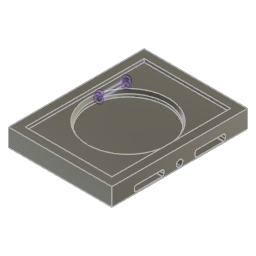
Plantillas_Taladrado (Autodesk Fusion 360 design; units mm, degrees)
Autodesk Fusion 360 part; units mm, degrees
note: some values were not read from the file. Set by a fixed rule: which sketch regions a step uses.
(part 1 of 4)
sketch "Boceto1" plane through (0, 0, 0) normal (0, 0, 1) x (1, 0, 0)
  line L0 (-350.383, -160) -> (-534, -160)
  line L1 (-455, -160) -> (-485, -160)
  line L2 (-349.3477, -167.8637) -> (-490.0029, -205.5522)
  line L3 (-513.132, -233.222) -> (-328.2758, -207.9962)
  line L4 (-333.1284, -237.9253) -> (-317, -237.9253) construction
  line L5 (246.2643, -265.6288) -> (-3.7357, -265.6288)
  line L6 (-3.7357, -235.6288) -> (246.2643, -235.6288)
  line L7 (246.2643, -235.6288) -> (246.2643, -265.6288)
  line L8 (-3.7357, -265.6288) -> (-3.7357, -235.6288)
  line L9 (-340.8744, -224.4717) -> (-532.4471, -275.8034)
  line L10 (-350.383, -160) -> (-534, -160)
  line L11 (-349.3477, -167.8637) -> (-490.0029, -205.5522)
  arc A0 (-334.1839, -233.9864) -> (-329.0577, -237.6835) centre (-329.3542, -232.6923) ccw
  line L12 (-517.6728, -197.507) -> (-517.6728, -229.2587)
  arc A1 (-496.8802, -195.3406) -> (-501.0926, -192.3911) centre (-500.7439, -196.3758) ccw
  line L13 (-326.1408, -237.5102) -> (-329.0577, -237.6835)
  line L14 (-497.7489, -192.0985) -> (-478.0528, -192.0985) construction
  line L15 (-501.0926, -192.3911) -> (-514.0215, -193.5222)
  arc A2 (-335.9754, -227.3001) -> (-340.8744, -224.4717) centre (-339.8392, -228.3354) ccw
  arc A3 (-534, -160) -> (-540, -166) centre (-534, -166) ccw
  line L16 (-497.7489, -192.0985) -> (-478.0528, -192.0985) construction
  line L17 (-334.1839, -233.9864) -> (-335.9754, -227.3001)
  arc A4 (-322.6085, -212.6538) -> (-328.2758, -207.9962) centre (-327.5997, -212.9503) ccw
  arc A5 (-326.1408, -237.5102) -> (-321.4461, -232.2225) centre (-326.4373, -232.519) ccw
  line L18 (-517.6728, -197.507) -> (-517.6728, -229.2587)
  circle A6 centre (-463, -175) radius 2.1
  arc A7 (-534, -160) -> (-540, -166) centre (-534, -166) ccw
  arc A8 (-349.3477, -167.8637) -> (-350.383, -160) centre (-350.383, -164) ccw
  arc A9 (-540, -270.0079) -> (-532.4471, -275.8034) centre (-534, -270.0079) ccw
  arc A10 (-335.9754, -227.3001) -> (-340.8744, -224.4717) centre (-339.8392, -228.3354) ccw
  arc A11 (-334.1839, -233.9864) -> (-329.0577, -237.6835) centre (-329.3542, -232.6923) ccw
  line L19 (-320, -160) -> (-304.7526, -160) construction
  line L20 (-494.9019, -202.7237) -> (-496.8802, -195.3406)
  line L21 (-540, -166) -> (-540, -270.0079)
  line L22 (-494.9019, -202.7237) -> (-496.8802, -195.3406)
  arc A12 (-494.9019, -202.7237) -> (-490.0029, -205.5522) centre (-491.0382, -201.6884) ccw
  line L23 (-322.6085, -212.6538) -> (-321.4461, -232.2225)
  line L24 (-501.0926, -192.3911) -> (-514.0215, -193.5222)
  arc A13 (-322.6085, -212.6538) -> (-328.2758, -207.9962) centre (-327.5997, -212.9503) ccw
  line L25 (-326.1408, -237.5102) -> (-329.0577, -237.6835)
  arc A14 (-514.0215, -193.5222) -> (-517.6728, -197.507) centre (-513.6728, -197.507) ccw
  arc A15 (-517.6728, -229.2587) -> (-513.132, -233.222) centre (-513.6728, -229.2587) ccw
  arc A16 (-494.9019, -202.7237) -> (-490.0029, -205.5522) centre (-491.0382, -201.6884) ccw
  arc A17 (-326.1408, -237.5102) -> (-321.4461, -232.2225) centre (-326.4373, -232.519) ccw
  line L26 (-322.6085, -212.6538) -> (-321.4461, -232.2225)
  arc A18 (-349.3477, -167.8637) -> (-350.383, -160) centre (-350.383, -164) ccw
  line L27 (-540, -166) -> (-540, -270.0079)
  arc A19 (-540, -270.0079) -> (-532.4471, -275.8034) centre (-534, -270.0079) ccw
  arc A20 (-496.8802, -195.3406) -> (-501.0926, -192.3911) centre (-500.7439, -196.3758) ccw
  circle A21 centre (-477, -175) radius 2.1
  arc A22 (-517.6728, -229.2587) -> (-513.132, -233.222) centre (-513.6728, -229.2587) ccw
  arc A23 (-514.0215, -193.5222) -> (-517.6728, -197.507) centre (-513.6728, -197.507) ccw
  line L28 (-513.132, -233.222) -> (-328.2758, -207.9962)
  line L29 (-340.8744, -224.4717) -> (-532.4471, -275.8034)
  line L30 (-334.1839, -233.9864) -> (-335.9754, -227.3001)
  line L31 (-525, -725) -> (-702.3195, -725)
  line L32 (1232.2, -850) -> (1286.175, -850)
  line L33 (-525, -547.6805) -> (-525, -573.0805)
  circle A24 centre (-525, -876.9195) radius 2.1
  circle A25 centre (-525, -573.0805) radius 2.1
  line L34 (263.0875, -557.9) -> (432.907, -557.9)
  line L35 (-525, -725) -> (-525, -902.3195)
  line L36 (0, -850) -> (53.975, -850)
  arc A26 (1023.0875, -697.7343) -> (828.975, -850) centre (1030.5875, -907.1583) ccw
  line L37 (248.0875, -627.75) -> (248.0875, -557.9)
  line L38 (432.907, -557.9) -> (263.0875, -557.9)
  line L39 (1030.5875, -627.75) -> (1023.0875, -627.75)
  line L40 (-347.6805, -725) -> (-373.0805, -725)
  line L41 (-525, -725) -> (-347.6805, -725)
  line L42 (1286.175, -850) -> (1207.907, -557.9)
  line L43 (775, -850) -> (853.268, -557.9)
  line L44 (263.0875, -557.9) -> (432.907, -557.9)
  line L45 (-347.6805, -725) -> (-296.8805, -725)
  line L46 (1038.0875, -627.75) -> (1038.0875, -697.7343)
  circle A27 centre (-373.0805, -725) radius 2.1
  line L47 (457.2, -850) -> (511.175, -850)
  circle A28 centre (-525, -725) radius 228.1195
  line L48 (511.175, -850) -> (510, -850)
  line L49 (511.175, -850) -> (457.2, -850)
  circle A29 centre (-676.9195, -725) radius 2.1
  line L50 (-702.3195, -725) -> (-676.9195, -725)
  line L51 (1030.5875, -627.75) -> (1038.0875, -627.75)
  arc A30 (457.2, -850) -> (53.975, -850) centre (255.5875, -907.1583) ccw
  line L52 (775, -850) -> (828.975, -850)
  line L53 (0, -850) -> (53.975, -850)
  line L54 (1286.175, -850) -> (1285, -850)
  line L55 (1207.907, -557.9) -> (1030.5875, -557.9)
  line L56 (0, -850) -> (78.268, -557.9)
  line L57 (263.0875, -557.9) -> (263.0875, -627.75)
  line L58 (1232.2, -850) -> (1286.175, -850)
  arc A31 (1232.2, -850) -> (1038.0875, -697.7343) centre (1030.5875, -907.1583) ccw
  line L59 (775, -850) -> (828.975, -850) construction
  line L60 (511.175, -850) -> (432.907, -557.9)
  line L61 (457.2, -850) -> (511.175, -850)
  line L62 (511.175, -850) -> (432.907, -557.9)
  line L63 (1286.175, -850) -> (1207.907, -557.9)
  line L64 (853.268, -557.9) -> (1207.907, -557.9)
  line L65 (-347.6805, -725) -> (-355.9463, -725)
  line L66 (1023.0875, -627.75) -> (1023.0875, -697.7343)
  line L67 (1286.175, -850) -> (1232.2, -850)
  line L68 (0, -850) -> (53.975, -850)
  line L69 (0, -850) -> (78.268, -557.9)
  line L70 (0, -850) -> (53.975, -850) construction
  line L71 (78.268, -557.9) -> (248.0875, -557.9)
  line L72 (853.268, -557.9) -> (1207.907, -557.9)
  line L73 (-525, -725) -> (-525, -547.6805)
  line L74 (78.268, -557.9) -> (248.0875, -557.9)
  line L75 (-525, -902.3195) -> (-525, -876.9195)
  line L76 (775, -850) -> (828.975, -850)
  line L77 (775, -850) -> (828.975, -850)
  line L78 (263.0875, -627.75) -> (248.0875, -627.75)
  line L79 (775, -850) -> (853.268, -557.9)
  line L80 (720, 610) -> (630, 610)
  line L81 (630, 610) -> (630, 415)
  line L82 (630, 415) -> (720, 415)
  line L83 (720, 610) -> (720, 415)
  line L84 (720, 415) -> (720, 610)
  line L85 (900, 595) -> (900, 700)
  line L86 (900, 700) -> (855, 700)
  line L87 (855, 655) -> (900, 655)
  circle A32 centre (855, 655) radius 17.5
  line L88 (870, 602.5) -> (900, 602.5)
  line L89 (840, 595) -> (840, 602.5)
  line L90 (900, 602.5) -> (900, 595)
  line L91 (870, 595) -> (870, 602.5)
  line L92 (900, 655) -> (900, 700)
  line L93 (900, 700) -> (810, 700)
  circle A33 centre (870, 602.5) radius 2.1
  line L94 (900, 595) -> (870, 595)
  line L95 (810, 602.5) -> (810, 595)
  line L96 (810, 700) -> (810, 595)
  line L97 (840, 602.5) -> (810, 602.5)
  line L98 (810, 595) -> (900, 595)
  line L99 (810, 595) -> (840, 595)
  circle A34 centre (840, 602.5) radius 2.1
  line L100 (810, 595) -> (810, 610)
  line L101 (855, 700) -> (855, 655)
  line L102 (-136.6668, 1350.1348) -> (-36.6668, 1350.1348)
  line L103 (-36.6668, 1350.1348) -> (-36.6668, 650.1348)
  line L104 (-36.6668, 650.1348) -> (-136.6668, 650.1348)
  line L105 (-136.6668, 650.1348) -> (-136.6668, 1350.1348)
  arc A35 (-699.3477, -167.8637) -> (-700.383, -160) centre (-700.383, -164) ccw
  arc A36 (-684.1839, -233.9864) -> (-679.0577, -237.6835) centre (-679.3542, -232.6923) ccw
  line L106 (-684.1839, -233.9864) -> (-685.9754, -227.3001)
  arc A37 (-685.9754, -227.3001) -> (-690.8744, -224.4717) centre (-689.8392, -228.3354) ccw
  line L107 (-676.1408, -237.5102) -> (-679.0577, -237.6835)
  line L108 (-672.6085, -212.6538) -> (-671.4461, -232.2225)
  line L109 (-863.132, -233.222) -> (-678.2758, -207.9962)
  line L110 (-690.8744, -224.4717) -> (-882.4471, -275.8034)
  arc A38 (-672.6085, -212.6538) -> (-678.2758, -207.9962) centre (-677.5997, -212.9503) ccw
  line L111 (-805, -160) -> (-835, -160)
  line L112 (-700.383, -160) -> (-884, -160)
  line L113 (-699.3477, -167.8637) -> (-840.0029, -205.5522)
  line L114 (-672.6085, -212.6538) -> (-671.4461, -232.2225)
  arc A39 (-672.6085, -212.6538) -> (-678.2758, -207.9962) centre (-677.5997, -212.9503) ccw
  line L115 (-700.383, -160) -> (-884, -160)
  line L116 (-690.8744, -224.4717) -> (-882.4471, -275.8034)
  line L117 (-863.132, -233.222) -> (-678.2758, -207.9962)
  line L118 (-851.0926, -192.3911) -> (-864.0215, -193.5222)
  arc A40 (-844.9019, -202.7237) -> (-840.0029, -205.5522) centre (-841.0382, -201.6884) ccw
  arc A41 (-676.1408, -237.5102) -> (-671.4461, -232.2225) centre (-676.4373, -232.519) ccw
  arc A42 (-890, -270.0079) -> (-882.4471, -275.8034) centre (-884, -270.0079) ccw
  line L119 (-844.9019, -202.7237) -> (-846.8802, -195.3406)
  arc A43 (-864.0215, -193.5222) -> (-867.6728, -197.507) centre (-863.6728, -197.507) ccw
  circle A44 centre (-827, -175) radius 2.1
  arc A45 (-867.6728, -229.2587) -> (-863.132, -233.222) centre (-863.6728, -229.2587) ccw
  arc A46 (-685.9754, -227.3001) -> (-690.8744, -224.4717) centre (-689.8392, -228.3354) ccw
  line L120 (-867.6728, -197.507) -> (-867.6728, -229.2587)
  line L121 (-890, -166) -> (-890, -270.0079)
  arc A47 (-884, -160) -> (-890, -166) centre (-884, -166) ccw
  arc A48 (-846.8802, -195.3406) -> (-851.0926, -192.3911) centre (-850.7439, -196.3758) ccw
  arc A49 (-867.6728, -229.2587) -> (-863.132, -233.222) centre (-863.6728, -229.2587) ccw
  arc A50 (-864.0215, -193.5222) -> (-867.6728, -197.507) centre (-863.6728, -197.507) ccw
  arc A51 (-846.8802, -195.3406) -> (-851.0926, -192.3911) centre (-850.7439, -196.3758) ccw
  line L122 (-847.7489, -192.0985) -> (-828.0528, -192.0985) construction
  line L123 (-867.6728, -197.507) -> (-867.6728, -229.2587)
  line L124 (-844.9019, -202.7237) -> (-846.8802, -195.3406)
  line L125 (-890, -166) -> (-890, -270.0079)
  arc A52 (-884, -160) -> (-890, -166) centre (-884, -166) ccw
  line L126 (-851.0926, -192.3911) -> (-864.0215, -193.5222)
  arc A53 (-844.9019, -202.7237) -> (-840.0029, -205.5522) centre (-841.0382, -201.6884) ccw
  arc A54 (-890, -270.0079) -> (-882.4471, -275.8034) centre (-884, -270.0079) ccw
  line L127 (-684.1839, -233.9864) -> (-685.9754, -227.3001)
  line L128 (-683.1284, -237.9253) -> (-667, -237.9253) construction
  arc A55 (-699.3477, -167.8637) -> (-700.383, -160) centre (-700.383, -164) ccw
  line L129 (-676.1408, -237.5102) -> (-679.0577, -237.6835)
  line L130 (-847.7489, -192.0985) -> (-828.0528, -192.0985) construction
  arc A56 (-676.1408, -237.5102) -> (-671.4461, -232.2225) centre (-676.4373, -232.519) ccw
  line L131 (-670, -160) -> (-654.7526, -160) construction
  line L132 (-699.3477, -167.8637) -> (-840.0029, -205.5522)
  arc A57 (-684.1839, -233.9864) -> (-679.0577, -237.6835) centre (-679.3542, -232.6923) ccw
  circle A58 centre (-813, -175) radius 2.1
  arc A59 (-349.3477, 82.1363) -> (-350.383, 90) centre (-350.383, 86) ccw
  arc A60 (-334.1839, 16.0136) -> (-329.0577, 12.3165) centre (-329.3542, 17.3077) ccw
  line L133 (-334.1839, 16.0136) -> (-335.9754, 22.6999)
  arc A61 (-335.9754, 22.6999) -> (-340.8744, 25.5283) centre (-339.8392, 21.6646) ccw
  line L134 (-326.1408, 12.4898) -> (-329.0577, 12.3165)
  line L135 (-322.6085, 37.3462) -> (-321.4461, 17.7775)
  line L136 (-513.132, 16.778) -> (-328.2758, 42.0038)
  line L137 (-340.8744, 25.5283) -> (-532.4471, -25.8034)
  arc A62 (-322.6085, 37.3462) -> (-328.2758, 42.0038) centre (-327.5997, 37.0497) ccw
  line L138 (-455, 90) -> (-485, 90)
  line L139 (-350.383, 90) -> (-534, 90)
  line L140 (-349.3477, 82.1363) -> (-490.0029, 44.4478)
  line L141 (-322.6085, 37.3462) -> (-321.4461, 17.7775)
  arc A63 (-322.6085, 37.3462) -> (-328.2758, 42.0038) centre (-327.5997, 37.0497) ccw
  line L142 (-350.383, 90) -> (-534, 90)
  line L143 (-340.8744, 25.5283) -> (-532.4471, -25.8034)
  line L144 (-513.132, 16.778) -> (-328.2758, 42.0038)
  line L145 (-501.0926, 57.6089) -> (-514.0215, 56.4778)
  arc A64 (-494.9019, 47.2763) -> (-490.0029, 44.4478) centre (-491.0382, 48.3116) ccw
  arc A65 (-326.1408, 12.4898) -> (-321.4461, 17.7775) centre (-326.4373, 17.481) ccw
  arc A66 (-540, -20.0079) -> (-532.4471, -25.8034) centre (-534, -20.0079) ccw
  line L146 (-494.9019, 47.2763) -> (-496.8802, 54.6594)
  arc A67 (-514.0215, 56.4778) -> (-517.6728, 52.493) centre (-513.6728, 52.493) ccw
  circle A68 centre (-477, 75) radius 2.1
  arc A69 (-517.6728, 20.7413) -> (-513.132, 16.778) centre (-513.6728, 20.7413) ccw
  arc A70 (-335.9754, 22.6999) -> (-340.8744, 25.5283) centre (-339.8392, 21.6646) ccw
  line L147 (-517.6728, 52.493) -> (-517.6728, 20.7413)
  line L148 (-540, 84) -> (-540, -20.0079)
  arc A71 (-534, 90) -> (-540, 84) centre (-534, 84) ccw
  arc A72 (-496.8802, 54.6594) -> (-501.0926, 57.6089) centre (-500.7439, 53.6242) ccw
  arc A73 (-517.6728, 20.7413) -> (-513.132, 16.778) centre (-513.6728, 20.7413) ccw
  arc A74 (-514.0215, 56.4778) -> (-517.6728, 52.493) centre (-513.6728, 52.493) ccw
  arc A75 (-496.8802, 54.6594) -> (-501.0926, 57.6089) centre (-500.7439, 53.6242) ccw
  line L149 (-497.7489, 57.9015) -> (-478.0528, 57.9015) construction
  line L150 (-517.6728, 52.493) -> (-517.6728, 20.7413)
  line L151 (-494.9019, 47.2763) -> (-496.8802, 54.6594)
  line L152 (-540, 84) -> (-540, -20.0079)
  arc A76 (-534, 90) -> (-540, 84) centre (-534, 84) ccw
  line L153 (-501.0926, 57.6089) -> (-514.0215, 56.4778)
  arc A77 (-494.9019, 47.2763) -> (-490.0029, 44.4478) centre (-491.0382, 48.3116) ccw
  arc A78 (-540, -20.0079) -> (-532.4471, -25.8034) centre (-534, -20.0079) ccw
  line L154 (-334.1839, 16.0136) -> (-335.9754, 22.6999)
  line L155 (-333.1284, 12.0747) -> (-317, 12.0747) construction
  arc A79 (-349.3477, 82.1363) -> (-350.383, 90) centre (-350.383, 86) ccw
  line L156 (-326.1408, 12.4898) -> (-329.0577, 12.3165)
  line L157 (-497.7489, 57.9015) -> (-478.0528, 57.9015) construction
  arc A80 (-326.1408, 12.4898) -> (-321.4461, 17.7775) centre (-326.4373, 17.481) ccw
  line L158 (-320, 90) -> (-304.7526, 90) construction
  line L159 (-349.3477, 82.1363) -> (-490.0029, 44.4478)
  arc A81 (-334.1839, 16.0136) -> (-329.0577, 12.3165) centre (-329.3542, 17.3077) ccw
  circle A82 centre (-463, 75) radius 2.1
  arc A83 (-699.3477, 82.1363) -> (-700.383, 90) centre (-700.383, 86) ccw
  arc A84 (-684.1839, 16.0136) -> (-679.0577, 12.3165) centre (-679.3542, 17.3077) ccw
  line L160 (-684.1839, 16.0136) -> (-685.9754, 22.6999)
  arc A85 (-685.9754, 22.6999) -> (-690.8744, 25.5283) centre (-689.8392, 21.6646) ccw
  line L161 (-676.1408, 12.4898) -> (-679.0577, 12.3165)
  line L162 (-672.6085, 37.3462) -> (-671.4461, 17.7775)
  line L163 (-863.132, 16.778) -> (-678.2758, 42.0038)
  line L164 (-690.8744, 25.5283) -> (-882.4471, -25.8034)
  arc A86 (-672.6085, 37.3462) -> (-678.2758, 42.0038) centre (-677.5997, 37.0497) ccw
  line L165 (-805, 90) -> (-835, 90)
  line L166 (-700.383, 90) -> (-884, 90)
  line L167 (-699.3477, 82.1363) -> (-840.0029, 44.4478)
  line L168 (-672.6085, 37.3462) -> (-671.4461, 17.7775)
  arc A87 (-672.6085, 37.3462) -> (-678.2758, 42.0038) centre (-677.5997, 37.0497) ccw
  line L169 (-700.383, 90) -> (-884, 90)
  line L170 (-690.8744, 25.5283) -> (-882.4471, -25.8034)
  line L171 (-863.132, 16.778) -> (-678.2758, 42.0038)
  line L172 (-851.0926, 57.6089) -> (-864.0215, 56.4778)
  arc A88 (-844.9019, 47.2763) -> (-840.0029, 44.4478) centre (-841.0382, 48.3116) ccw
  arc A89 (-676.1408, 12.4898) -> (-671.4461, 17.7775) centre (-676.4373, 17.481) ccw
  arc A90 (-890, -20.0079) -> (-882.4471, -25.8034) centre (-884, -20.0079) ccw
  line L173 (-844.9019, 47.2763) -> (-846.8802, 54.6594)
  arc A91 (-864.0215, 56.4778) -> (-867.6728, 52.493) centre (-863.6728, 52.493) ccw
  circle A92 centre (-827, 75) radius 2.1
  arc A93 (-867.6728, 20.7413) -> (-863.132, 16.778) centre (-863.6728, 20.7413) ccw
  arc A94 (-685.9754, 22.6999) -> (-690.8744, 25.5283) centre (-689.8392, 21.6646) ccw
  line L174 (-867.6728, 52.493) -> (-867.6728, 20.7413)
  line L175 (-890, 84) -> (-890, -20.0079)
  arc A95 (-884, 90) -> (-890, 84) centre (-884, 84) ccw
  arc A96 (-846.8802, 54.6594) -> (-851.0926, 57.6089) centre (-850.7439, 53.6242) ccw
  arc A97 (-867.6728, 20.7413) -> (-863.132, 16.778) centre (-863.6728, 20.7413) ccw
  arc A98 (-864.0215, 56.4778) -> (-867.6728, 52.493) centre (-863.6728, 52.493) ccw
  arc A99 (-846.8802, 54.6594) -> (-851.0926, 57.6089) centre (-850.7439, 53.6242) ccw
  line L176 (-847.7489, 57.9015) -> (-828.0528, 57.9015) construction
  line L177 (-867.6728, 52.493) -> (-867.6728, 20.7413)
  line L178 (-844.9019, 47.2763) -> (-846.8802, 54.6594)
  line L179 (-890, 84) -> (-890, -20.0079)
  arc A100 (-884, 90) -> (-890, 84) centre (-884, 84) ccw
  line L180 (-851.0926, 57.6089) -> (-864.0215, 56.4778)
  arc A101 (-844.9019, 47.2763) -> (-840.0029, 44.4478) centre (-841.0382, 48.3116) ccw
  arc A102 (-890, -20.0079) -> (-882.4471, -25.8034) centre (-884, -20.0079) ccw
  line L181 (-684.1839, 16.0136) -> (-685.9754, 22.6999)
  line L182 (-683.1284, 12.0747) -> (-667, 12.0747) construction
  arc A103 (-699.3477, 82.1363) -> (-700.383, 90) centre (-700.383, 86) ccw
  line L183 (-676.1408, 12.4898) -> (-679.0577, 12.3165)
  line L184 (-847.7489, 57.9015) -> (-828.0528, 57.9015) construction
  arc A104 (-676.1408, 12.4898) -> (-671.4461, 17.7775) centre (-676.4373, 17.481) ccw
  line L185 (-670, 90) -> (-654.7526, 90) construction
  line L186 (-699.3477, 82.1363) -> (-840.0029, 44.4478)
  arc A105 (-684.1839, 16.0136) -> (-679.0577, 12.3165) centre (-679.3542, 17.3077) ccw
  circle A106 centre (-813, 75) radius 2.1
  line L187 (246.2643, 34.3712) -> (-3.7357, 34.3712)
  line L188 (-3.7357, 64.3712) -> (246.2643, 64.3712)
  line L189 (-3.7357, 34.3712) -> (-3.7357, 64.3712)
  line L190 (246.2643, 64.3712) -> (246.2643, 34.3712)
  line L191 (1420, 595) -> (1420, 602.5)
  line L192 (1270, 610) -> (1180, 610)
  line L193 (1405, 700) -> (1405, 655)
  line L194 (1450, 595) -> (1420, 595)
  line L195 (1450, 700) -> (1405, 700)
  line L196 (1450, 595) -> (1450, 700)
  line L197 (1360, 602.5) -> (1360, 595)
  line L198 (1360, 595) -> (1360, 610)
  circle A107 centre (1420, 602.5) radius 2.1
  line L199 (1180, 610) -> (1180, 415)
  line L200 (1390, 602.5) -> (1360, 602.5)
  line L201 (1180, 415) -> (1270, 415)
  line L202 (1420, 602.5) -> (1450, 602.5)
  line L203 (1405, 655) -> (1450, 655)
  line L204 (1270, 415) -> (1270, 610)
  circle A108 centre (1390, 602.5) radius 2.1
  line L205 (1450, 700) -> (1360, 700)
  line L206 (1450, 655) -> (1450, 700)
  line L207 (1360, 595) -> (1450, 595)
  line L208 (1450, 602.5) -> (1450, 595)
  line L209 (1270, 610) -> (1270, 415)
  circle A109 centre (1405, 655) radius 17.5
  line L210 (1360, 700) -> (1360, 595)
  line L211 (1390, 595) -> (1390, 602.5)
  line L212 (1360, 595) -> (1390, 595)
  line L213 (870, 1045) -> (870, 1052.5)
  line L214 (720, 1060) -> (630, 1060)
  line L215 (855, 1150) -> (855, 1105)
  line L216 (900, 1045) -> (870, 1045)
  line L217 (900, 1150) -> (855, 1150)
  line L218 (900, 1045) -> (900, 1150)
  line L219 (810, 1052.5) -> (810, 1045)
  line L220 (810, 1045) -> (810, 1060)
  circle A110 centre (870, 1052.5) radius 2.1
  line L221 (630, 1060) -> (630, 865)
  line L222 (840, 1052.5) -> (810, 1052.5)
  line L223 (630, 865) -> (720, 865)
  line L224 (870, 1052.5) -> (900, 1052.5)
  line L225 (855, 1105) -> (900, 1105)
  line L226 (720, 865) -> (720, 1060)
  circle A111 centre (840, 1052.5) radius 2.1
  line L227 (900, 1150) -> (810, 1150)
  line L228 (900, 1105) -> (900, 1150)
  line L229 (810, 1045) -> (900, 1045)
  line L230 (900, 1052.5) -> (900, 1045)
  line L231 (720, 1060) -> (720, 865)
  circle A112 centre (855, 1105) radius 17.5
  line L232 (810, 1150) -> (810, 1045)
  line L233 (840, 1045) -> (840, 1052.5)
  line L234 (810, 1045) -> (840, 1045)
  line L235 (1420, 1045) -> (1420, 1052.5)
  line L236 (1270, 1060) -> (1180, 1060)
  line L237 (1405, 1150) -> (1405, 1105)
  line L238 (1450, 1045) -> (1420, 1045)
  line L239 (1450, 1150) -> (1405, 1150)
  line L240 (1450, 1045) -> (1450, 1150)
  line L241 (1360, 1052.5) -> (1360, 1045)
  line L242 (1360, 1045) -> (1360, 1060)
  circle A113 centre (1420, 1052.5) radius 2.1
  line L243 (1180, 1060) -> (1180, 865)
  line L244 (1390, 1052.5) -> (1360, 1052.5)
  line L245 (1180, 865) -> (1270, 865)
  line L246 (1420, 1052.5) -> (1450, 1052.5)
  line L247 (1405, 1105) -> (1450, 1105)
  line L248 (1270, 865) -> (1270, 1060)
  circle A114 centre (1390, 1052.5) radius 2.1
  line L249 (1450, 1150) -> (1360, 1150)
  line L250 (1450, 1105) -> (1450, 1150)
  line L251 (1360, 1045) -> (1450, 1045)
  line L252 (1450, 1052.5) -> (1450, 1045)
  line L253 (1270, 1060) -> (1270, 865)
  circle A115 centre (1405, 1105) radius 17.5
  line L254 (1360, 1150) -> (1360, 1045)
  line L255 (1390, 1045) -> (1390, 1052.5)
  line L256 (1360, 1045) -> (1390, 1045)
  line L257 (2613.3332, 1350.1348) -> (3108.308, 855.1601)
  line L258 (3037.5973, 784.4494) -> (2542.6226, 1279.4241)
  line L259 (2542.6226, 1279.4241) -> (2613.3332, 1350.1348)
  line L260 (3108.308, 855.1601) -> (3037.5973, 784.4494)
  line L261 (2500, 1375) -> (3200, 1375)
  line L262 (3200, 1375) -> (3200, 675)
  line L263 (3200, 675) -> (2500, 675)
  line L264 (2500, 675) -> (2500, 1375)
  line L265 (3150, -275) -> (2500, -275)
  line L266 (3150, 375) -> (3150, -275)
  line L267 (2500, -275) -> (2500, 375)
  line L268 (2500, 375) -> (3150, 375)
  line L269 (2830.5875, 72.25) -> (2838.0875, 72.25)
  line L270 (2575, -150) -> (2628.975, -150)
  line L271 (2653.268, 142.1) -> (3007.907, 142.1)
  line L272 (3086.175, -150) -> (3085, -150)
  line L273 (2575, -150) -> (2628.975, -150)
  line L274 (2653.268, 142.1) -> (3007.907, 142.1)
  line L275 (3032.2, -150) -> (3086.175, -150)
  line L276 (3007.907, 142.1) -> (2830.5875, 142.1)
  line L277 (2830.5875, 72.25) -> (2823.0875, 72.25)
  line L278 (3086.175, -150) -> (3007.907, 142.1)
  arc A116 (3032.2, -150) -> (2838.0875, 2.2657) centre (2830.5875, -207.1583) ccw
  line L279 (2838.0875, 72.25) -> (2838.0875, 2.2657)
  line L280 (2575, -150) -> (2653.268, 142.1)
  line L281 (3086.175, -150) -> (3032.2, -150)
  line L282 (3032.2, -150) -> (3086.175, -150)
  line L283 (2575, -150) -> (2628.975, -150)
  line L284 (3086.175, -150) -> (3007.907, 142.1)
  line L285 (2575, -150) -> (2653.268, 142.1)
  line L286 (2575, -150) -> (2628.975, -150) construction
  arc A117 (2823.0875, 2.2657) -> (2628.975, -150) centre (2830.5875, -207.1583) ccw
  line L287 (2823.0875, 72.25) -> (2823.0875, 2.2657)
  line L288 (2800, -2100) -> (5200, -2100)
  line L289 (5200, -2100) -> (5200, -3900)
  line L290 (5200, -3900) -> (2800, -3900)
  line L291 (2800, -3900) -> (2800, -2100)
  line L292 (2800, -2100) -> (3500, -2100)
  line L293 (3500, -2100) -> (3500, -3200)
  line L294 (3500, -3200) -> (2800, -3200)
  line L295 (2800, -3200) -> (2800, -2100)
  line L296 (3500, -2100) -> (4200, -2100)
  line L297 (4200, -3200) -> (3500, -3200)
  line L298 (3500, -3200) -> (3500, -2100)
  line L299 (4200, -2100) -> (4200, -3200)
  line L300 (4200, -2100) -> (4900, -2100)
  line L301 (4900, -3200) -> (4200, -3200)
  line L302 (4200, -3200) -> (4200, -2100)
  line L303 (4900, -2100) -> (4900, -3200)
  line L304 (3900, -3200) -> (3900, -3900)
  line L305 (2800, -3900) -> (2800, -3200)
  line L306 (2800, -3200) -> (3900, -3200)
  line L307 (3900, -3900) -> (2800, -3900)
  line L308 (5000, -3200) -> (5000, -3900)
  line L309 (3900, -3900) -> (3900, -3200)
  line L310 (3900, -3200) -> (5000, -3200)
  line L311 (5000, -3900) -> (3900, -3900)
  line L312 (-36.6668, 650.1348) -> (-136.6668, 650.1348)
  line L313 (-136.6668, 650.1348) -> (-136.6668, 1350.1348)
  line L314 (-36.6668, 1350.1348) -> (-36.6668, 650.1348)
  line L315 (-136.6668, 1350.1348) -> (-36.6668, 1350.1348)
  line L316 (-347.6805, -725) -> (-355.9463, -725)
  circle A118 centre (-525, -573.0805) radius 2.1
  line L317 (-525, -725) -> (-347.6805, -725)
  line L318 (-525, -547.6805) -> (-525, -573.0805)
  circle A119 centre (-676.9195, -725) radius 2.1
  circle A120 centre (-525, -725) radius 228.1195
  line L319 (-525, -725) -> (-525, -547.6805)
  circle A121 centre (-373.0805, -725) radius 2.1
  line L320 (-347.6805, -725) -> (-373.0805, -725)
  line L321 (-702.3195, -725) -> (-676.9195, -725)
  line L322 (-525, -725) -> (-525, -902.3195)
  line L323 (-525, -902.3195) -> (-525, -876.9195)
  circle A122 centre (-525, -876.9195) radius 2.1
  line L324 (-525, -725) -> (-702.3195, -725)
  line L325 (-347.6805, -725) -> (-296.8805, -725)
  line L326 (-1200, -1600) -> (-590.4, -1600)
  line L327 (-590.4, -1600) -> (-590.4, -2400)
  line L328 (-590.4, -2400) -> (-1200, -2400)
  line L329 (-1200, -2400) -> (-1200, -1600)
  line L330 (-525, -725) -> (-347.6805, -725)
  line L331 (-347.6805, -725) -> (-373.0805, -725)
  line L332 (-525, -725) -> (-525, -902.3195)
  line L333 (-525, -725) -> (-702.3195, -725)
  line L334 (-525, -547.6805) -> (-525, -573.0805)
  line L335 (-525, -902.3195) -> (-525, -876.9195)
  circle A123 centre (-676.9195, -725) radius 2.1
  circle A124 centre (-525, -573.0805) radius 2.1
  line L336 (-525, -725) -> (-525, -902.3195)
  line L337 (-525, -725) -> (-525, -547.6805)
  circle A125 centre (-525, -876.9195) radius 2.1
  line L338 (-525, -725) -> (-525, -547.6805)
  line L339 (-702.3195, -725) -> (-676.9195, -725)
  line L340 (-525, -547.6805) -> (-525, -573.0805)
  line L341 (-347.6805, -725) -> (-296.8805, -725)
  line L342 (-347.6805, -725) -> (-355.9463, -725)
  line L343 (-347.6805, -725) -> (-373.0805, -725)
  line L344 (-347.6805, -725) -> (-355.9463, -725)
  line L345 (-347.6805, -725) -> (-296.8805, -725)
  line L346 (-525, -725) -> (-347.6805, -725)
  circle A126 centre (-525, -725) radius 228.1195
  circle A127 centre (-373.0805, -725) radius 2.1
  circle A128 centre (-373.0805, -725) radius 2.1
  circle A129 centre (-525, -573.0805) radius 2.1
  circle A130 centre (-525, -725) radius 228.1195
  circle A131 centre (-676.9195, -725) radius 2.1
  line L347 (-525, -725) -> (-702.3195, -725)
  circle A132 centre (-525, -876.9195) radius 2.1
  line L348 (-525, -902.3195) -> (-525, -876.9195)
  line L349 (-702.3195, -725) -> (-676.9195, -725)
  line L350 (-347.6805, -725) -> (-373.0805, -725)
  circle A133 centre (-373.0805, -725) radius 2.1
  line L351 (-347.6805, -725) -> (-373.0805, -725)
  circle A134 centre (-373.0805, -725) radius 2.1
  circle A135 centre (-373.0805, -725) radius 2.1
  circle A136 centre (-525, -725) radius 228.1195
  line L352 (-347.6805, -725) -> (-296.8805, -725)
  line L353 (-347.6805, -725) -> (-355.9463, -725)
  circle A137 centre (-373.0805, -725) radius 2.1
  line L354 (-525, -725) -> (-347.6805, -725)
  line L355 (-347.6805, -725) -> (-296.8805, -725)
  line L356 (-347.6805, -725) -> (-373.0805, -725)
  line L357 (-347.6805, -725) -> (-296.8805, -725)
  line L358 (-347.6805, -725) -> (-355.9463, -725)
  line L359 (-347.6805, -725) -> (-355.9463, -725)
  line L360 (-525, -725) -> (-347.6805, -725)
  line L361 (-347.6805, -725) -> (-296.8805, -725)
  line L362 (-347.6805, -725) -> (-373.0805, -725)
  line L363 (-347.6805, -725) -> (-355.9463, -725)
  line L364 (-525, -725) -> (-347.6805, -725)
  line L365 (-525, -547.6805) -> (-525, -573.0805)
  circle A138 centre (-676.9195, -725) radius 2.1
  line L366 (-525, -725) -> (-702.3195, -725)
  circle A139 centre (-676.9195, -725) radius 2.1
  line L367 (-525, -902.3195) -> (-525, -876.9195)
  line L368 (-525, -725) -> (-525, -547.6805)
  line L369 (-525, -725) -> (-702.3195, -725)
  line L370 (-702.3195, -725) -> (-676.9195, -725)
  line L371 (-525, -725) -> (-525, -547.6805)
  line L372 (-525, -725) -> (-702.3195, -725)
  circle A140 centre (-676.9195, -725) radius 2.1
  circle A141 centre (-525, -725) radius 228.1195
  line L373 (-702.3195, -725) -> (-676.9195, -725)
  circle A142 centre (-525, -876.9195) radius 2.1
  line L374 (-525, -725) -> (-525, -902.3195)
  line L375 (-702.3195, -725) -> (-676.9195, -725)
  circle A143 centre (-676.9195, -725) radius 2.1
  line L376 (-525, -902.3195) -> (-525, -876.9195)
  line L377 (-702.3195, -725) -> (-676.9195, -725)
  circle A144 centre (-525, -876.9195) radius 2.1
  line L378 (-525, -725) -> (-525, -902.3195)
  line L379 (-525, -725) -> (-702.3195, -725)
  circle A145 centre (-525, -573.0805) radius 2.1
  circle A146 centre (-525, -573.0805) radius 2.1
  circle A147 centre (-525, -725) radius 228.1195
  circle A148 centre (-525, -725) radius 228.1195
  line L380 (-525, -725) -> (-525, -547.6805)
  line L381 (-525, -725) -> (-525, -902.3195)
  line L382 (-525, -547.6805) -> (-525, -573.0805)
  line L383 (-525, -902.3195) -> (-525, -876.9195)
  line L384 (-525, -547.6805) -> (-525, -573.0805)
  circle A149 centre (-525, -573.0805) radius 2.1
  line L385 (-525, -725) -> (-347.6805, -725)
  circle A150 centre (-525, -876.9195) radius 2.1
  line L386 (-525, -725) -> (-525, -902.3195)
  circle A151 centre (-525, -876.9195) radius 2.1
  line L387 (-525, -902.3195) -> (-525, -876.9195)
  circle A152 centre (-525, -573.0805) radius 2.1
  line L388 (-525, -547.6805) -> (-525, -573.0805)
  line L389 (-525, -725) -> (-525, -547.6805)
  line L390 (-347.6805, -725) -> (-373.0805, -725)
  circle A153 centre (-525, -725) radius 228.1195
  line L391 (-347.6805, -725) -> (-355.9463, -725)
  line L392 (-347.6805, -725) -> (-355.9463, -725)
  line L393 (-347.6805, -725) -> (-355.9463, -725)
  line L394 (-347.6805, -725) -> (-373.0805, -725)
  line L395 (-347.6805, -725) -> (-296.8805, -725)
  line L396 (-347.6805, -725) -> (-355.9463, -725)
  line L397 (-347.6805, -725) -> (-296.8805, -725)
  line L398 (-347.6805, -725) -> (-373.0805, -725)
  circle A154 centre (-525, -573.0805) radius 2.1
  line L399 (-525, -725) -> (-702.3195, -725)
  line L400 (-525, -725) -> (-702.3195, -725)
  circle A155 centre (-525, -573.0805) radius 2.1
  line L401 (-525, -902.3195) -> (-525, -876.9195)
  line L402 (-525, -725) -> (-702.3195, -725)
  line L403 (-525, -547.6805) -> (-525, -573.0805)
  circle A156 centre (-525, -573.0805) radius 2.1
  line L404 (-525, -547.6805) -> (-525, -573.0805)
  line L405 (-525, -547.6805) -> (-525, -573.0805)
  circle A157 centre (-525, -573.0805) radius 2.1
  line L406 (-525, -725) -> (-525, -902.3195)
  line L407 (-525, -902.3195) -> (-525, -876.9195)
  circle A158 centre (-525, -876.9195) radius 2.1
  circle A159 centre (-525, -876.9195) radius 2.1
  circle A160 centre (-525, -876.9195) radius 2.1
  line L408 (-525, -547.6805) -> (-525, -573.0805)
  line L409 (-525, -547.6805) -> (-525, -573.0805)
  line L410 (-525, -547.6805) -> (-525, -573.0805)
  circle A161 centre (-525, -573.0805) radius 2.1
  line L411 (-525, -547.6805) -> (-525, -573.0805)
  circle A162 centre (-525, -573.0805) radius 2.1
  line L412 (-525, -547.6805) -> (-525, -573.0805)
  circle A163 centre (-525, -573.0805) radius 2.1
  circle A164 centre (-525, -573.0805) radius 2.1
  circle A165 centre (-676.9195, -725) radius 2.1
  line L413 (-525, -725) -> (-347.6805, -725)
  line L414 (-525, -725) -> (-347.6805, -725)
  circle A166 centre (-676.9195, -725) radius 2.1
  circle A167 centre (-676.9195, -725) radius 2.1
  line L415 (-702.3195, -725) -> (-676.9195, -725)
  line L416 (-702.3195, -725) -> (-676.9195, -725)
  line L417 (-525, -725) -> (-347.6805, -725)
  line L418 (-702.3195, -725) -> (-676.9195, -725)
  line L419 (-702.3195, -725) -> (-676.9195, -725)
  line L420 (-702.3195, -725) -> (-676.9195, -725)
  circle A168 centre (-676.9195, -725) radius 2.1
  circle A169 centre (-676.9195, -725) radius 2.1
  circle A170 centre (-676.9195, -725) radius 2.1
  circle A171 centre (-676.9195, -725) radius 2.1
  circle A172 centre (-676.9195, -725) radius 2.1
  line L421 (-702.3195, -725) -> (-676.9195, -725)
  line L422 (-702.3195, -725) -> (-676.9195, -725)
  line L423 (-347.6805, -725) -> (-355.9463, -725)
  line L424 (-347.6805, -725) -> (-373.0805, -725)
  line L425 (-347.6805, -725) -> (-296.8805, -725)
  line L426 (-347.6805, -725) -> (-296.8805, -725)
  line L427 (-525, -902.3195) -> (-525, -876.9195)
  circle A173 centre (-525, -725) radius 228.1195
  line L428 (-525, -725) -> (-525, -902.3195)
  line L429 (-525, -725) -> (-525, -902.3195)
  line L430 (-525, -725) -> (-525, -547.6805)
  line L431 (-525, -725) -> (-347.6805, -725)
  line L432 (-525, -725) -> (-525, -547.6805)
  line L433 (-525, -725) -> (-525, -547.6805)
  line L434 (-525, -725) -> (-525, -547.6805)
  circle A174 centre (-525, -725) radius 228.1195
  line L435 (-525, -725) -> (-702.3195, -725)
  circle A175 centre (-525, -725) radius 228.1195
  circle A176 centre (-525, -876.9195) radius 2.1
  line L436 (-525, -725) -> (-525, -547.6805)
  line L437 (-525, -725) -> (-347.6805, -725)
  line L438 (-525, -725) -> (-525, -902.3195)
  circle A177 centre (-525, -725) radius 228.1195
  line L439 (-525, -725) -> (-702.3195, -725)
  line L440 (-525, -902.3195) -> (-525, -876.9195)
  line L441 (-525, -725) -> (-702.3195, -725)
  line L442 (-525, -725) -> (-347.6805, -725)
  line L443 (-525, -725) -> (-525, -902.3195)
  circle A178 centre (-525, -876.9195) radius 2.1
  line L444 (-702.3195, -725) -> (-676.9195, -725)
  circle A179 centre (-525, -725) radius 228.1195
  circle A180 centre (-525, -725) radius 228.1195
  line L445 (-525, -725) -> (-347.6805, -725)
  line L446 (-525, -725) -> (-525, -902.3195)
  circle A181 centre (-525, -876.9195) radius 2.1
  line L447 (-525, -725) -> (-702.3195, -725)
  line L448 (-525, -902.3195) -> (-525, -876.9195)
  circle A182 centre (-525, -725) radius 228.1195
  line L449 (-525, -902.3195) -> (-525, -876.9195)
  line L450 (-525, -725) -> (-702.3195, -725)
  line L451 (-525, -725) -> (-525, -547.6805)
  circle A183 centre (-525, -876.9195) radius 2.1
  line L452 (-525, -725) -> (-525, -902.3195)
  line L453 (-525, -725) -> (-525, -902.3195)
  line L454 (-525, -725) -> (-525, -547.6805)
  line L455 (-525, -902.3195) -> (-525, -876.9195)
  circle A184 centre (-525, -876.9195) radius 2.1
  line L456 (-525, -902.3195) -> (-525, -876.9195)
  line L457 (-525, -725) -> (-525, -547.6805)
  circle A185 centre (-373.0805, -725) radius 2.1
  line L458 (-347.6805, -725) -> (-355.9463, -725)
  circle A186 centre (-373.0805, -725) radius 2.1
  circle A187 centre (-373.0805, -725) radius 2.1
  circle A188 centre (-373.0805, -725) radius 2.1
  circle A189 centre (-373.0805, -725) radius 2.1
  line L459 (-347.6805, -725) -> (-373.0805, -725)
  line L460 (-347.6805, -725) -> (-296.8805, -725)
  line L461 (-347.6805, -725) -> (-296.8805, -725)
  line L462 (-347.6805, -725) -> (-373.0805, -725)
  line L463 (-347.6805, -725) -> (-373.0805, -725)
  line L464 (-347.6805, -725) -> (-296.8805, -725)
  line L465 (-347.6805, -725) -> (-373.0805, -725)
  line L466 (-347.6805, -725) -> (-296.8805, -725)
  line L467 (-525, -725) -> (-347.6805, -725)
  line L468 (-347.6805, -725) -> (-355.9463, -725)
  line L469 (-347.6805, -725) -> (-355.9463, -725)
  circle A190 centre (-373.0805, -725) radius 2.1
  circle A191 centre (-373.0805, -725) radius 2.1
  circle A192 centre (-373.0805, -725) radius 2.1
  point P0 (-322.9285, -207.2665)
  point P1 (-337.0107, -223.4364)
  point P2 (-517.6728, -193.8417)
  point P3 (-321.1496, -237.2137)
  point P4 (-517.6728, -233.8417)
  point P5 (-493.8666, -206.5874)
  point P6 (-322.9285, -207.2665)
  point P7 (-517.6728, -233.8417)
  point P8 (-337.0107, -223.4364)
  point P9 (-540, -160)
  point P10 (-320, -160)
  point P11 (-517.6728, -193.8417)
  point P12 (-321.1496, -237.2137)
  point P13 (-493.8666, -206.5874)
  point P14 (-540, -160)
  point P15 (900, 700)
  point P16 (-687.0107, -223.4364)
  point P17 (-672.9285, -207.2665)
  point P18 (-671.1496, -237.2137)
  point P19 (-867.6728, -193.8417)
  point P20 (-867.6728, -233.8417)
  point P21 (-867.6728, -193.8417)
  point P22 (-687.0107, -223.4364)
  point P23 (-890, -160)
  point P24 (-670, -160)
  point P25 (-671.1496, -237.2137)
  point P26 (-890, -160)
  point P27 (-843.8666, -206.5874)
  point P28 (-843.8666, -206.5874)
  point P29 (-672.9285, -207.2665)
  point P30 (-867.6728, -233.8417)
  point P31 (-337.0107, 26.5636)
  point P32 (-322.9285, 42.7335)
  point P33 (-321.1496, 12.7863)
  point P34 (-517.6728, 56.1583)
  point P35 (-517.6728, 16.1583)
  point P36 (-517.6728, 56.1583)
  point P37 (-337.0107, 26.5636)
  point P38 (-540, 90)
  point P39 (-320, 90)
  point P40 (-321.1496, 12.7863)
  point P41 (-540, 90)
  point P42 (-493.8666, 43.4126)
  point P43 (-493.8666, 43.4126)
  point P44 (-322.9285, 42.7335)
  point P45 (-517.6728, 16.1583)
  point P46 (-687.0107, 26.5636)
  point P47 (-672.9285, 42.7335)
  point P48 (-671.1496, 12.7863)
  point P49 (-867.6728, 56.1583)
  point P50 (-867.6728, 16.1583)
  point P51 (-867.6728, 56.1583)
  point P52 (-687.0107, 26.5636)
  point P53 (-890, 90)
  point P54 (-670, 90)
  point P55 (-671.1496, 12.7863)
  point P56 (-890, 90)
  point P57 (-843.8666, 43.4126)
  point P58 (-843.8666, 43.4126)
  point P59 (-672.9285, 42.7335)
  point P60 (-867.6728, 16.1583)
  point P61 (1450, 700)
  point P62 (900, 1150)
  point P63 (1450, 1150)
  dimension "d142" = 250
  dimension "d143" = 30
  dimension "d899" = 220
  dimension "d900" = 165
  dimension "d901" = 180
  dimension "d902" = 15
  dimension "d903" = 175
  dimension "d907" = 30
  dimension "d908" = 12
  dimension "d909" = 105
  dimension "d910" = 15
  dimension "d911" = 40
  dimension "d913" = 6
  dimension "d914" = 4
  dimension "d915" = 4
  dimension "d919" = 4
  dimension "d920" = 5
  dimension "d923" = 220
  dimension "d927" = 20
  dimension "d928" = 30
  dimension "d933" = 6
  dimension "d937" = 4
  dimension "d938" = 4
  dimension "d939" = 4
  dimension "d941" = 5
  dimension "d942" = 5
  dimension "d943" = 5
  dimension "d949" = 4.2
  dimension "d950" = 4.2
  dimension "d144" = 511.175
  dimension "d147" = 354.6391
  dimension "d148" = 511.175
  dimension "d149" = 75
  dimension "d150" = 354.6391
  dimension "d151" = 53.975
  dimension "d152" = 53.975
  dimension "d153" = 511.175
  dimension "d155" = 354.6391
  dimension "d156" = 511.175
  dimension "d157" = 75
  dimension "d158" = 354.6391
  dimension "d159" = 53.975
  dimension "d160" = 53.975
  dimension "d161" = 177.3195
  dimension "d162" = 69.85
  dimension "d163" = 15
  dimension "d164" = 69.85
  dimension "d165" = 7.5
  dimension "d166" = 7.5
  dimension "d167" = 177.3195
  dimension "d168" = 177.3195
  dimension "d169" = 177.3195
  dimension "d170" = 177.3195
  dimension "d171" = 25.4
  dimension "d172" = 25.4
  dimension "d173" = 25.4
  dimension "d174" = 25.4
  dimension "d175" = 4.2
  dimension "d176" = 4.2
  dimension "d177" = 4.2
  dimension "d178" = 4.2
  dimension "d179" = 50.8
  dimension "d218" = 90
  dimension "d219" = 105
  dimension "d220" = 45
  dimension "d221" = 45
  dimension "d222" = 35
  dimension "d226" = 90
  dimension "d227" = 195
  dimension "d381" = 100
  dimension "d382" = 700
  dimension "d383" = 35
  dimension "d384" = 45
  dimension "d385" = 210
  dimension "d386" = 135
  dimension "d387" = 105
  dimension "d388" = 15
  dimension "d389" = 15
  dimension "d390" = 27.5
  dimension "d391" = 7.5
  dimension "d392" = 42.5
  dimension "d393" = 30
  dimension "d394" = 4.2
  dimension "d395" = 7.5
  dimension "d396" = 25
  dimension "d397" = 30
  dimension "d400" = 165
  dimension "d401" = 105
  dimension "d402" = 15
  dimension "d403" = 27.5
  dimension "d404" = 7.5
  dimension "d405" = 42.5
  dimension "d406" = 30
  dimension "d408" = 7.5
  dimension "d409" = 25
  dimension "d410" = 30
  dimension "d413" = 45
  dimension "d414" = 210
  dimension "d415" = 135
  dimension "d416" = 105
  dimension "d417" = 15
  dimension "d418" = 15
  dimension "d419" = 27.5
  dimension "d420" = 7.5
  dimension "d421" = 42.5
  dimension "d422" = 30
  dimension "d424" = 7.5
  dimension "d425" = 25
  dimension "d426" = 30
  dimension "d429" = 165
  dimension "d430" = 105
  dimension "d431" = 15
  dimension "d432" = 27.5
  dimension "d433" = 7.5
  dimension "d434" = 42.5
  dimension "d435" = 30
  dimension "d437" = 7.5
  dimension "d438" = 25
  dimension "d439" = 30
  dimension "d442" = 165
  dimension "d443" = 105
  dimension "d444" = 15
  dimension "d445" = 27.5
  dimension "d446" = 7.5
  dimension "d447" = 42.5
  dimension "d448" = 30
  dimension "d450" = 7.5
  dimension "d451" = 25
  dimension "d452" = 30
  dimension "d455" = 45
  dimension "d456" = 210
  dimension "d457" = 135
  dimension "d458" = 105
  dimension "d459" = 15
  dimension "d460" = 15
  dimension "d461" = 27.5
  dimension "d462" = 7.5
  dimension "d463" = 42.5
  dimension "d464" = 30
  dimension "d466" = 7.5
  dimension "d467" = 25
  dimension "d468" = 30
  dimension "d471" = 165
  dimension "d472" = 105
  dimension "d473" = 15
  dimension "d474" = 27.5
  dimension "d475" = 7.5
  dimension "d476" = 42.5
  dimension "d477" = 30
  dimension "d479" = 7.5
  dimension "d480" = 25
  dimension "d481" = 30
  dimension "d484" = 15
  dimension "d485" = 45
  dimension "d486" = 210
  dimension "d487" = 135
  dimension "d488" = 105
  dimension "d489" = 15
  dimension "d490" = 15
  dimension "d491" = 27.5
  dimension "d492" = 7.5
  dimension "d493" = 42.5
  dimension "d494" = 30
  dimension "d496" = 7.5
  dimension "d497" = 25
  dimension "d498" = 30
  dimension "d501" = 105
  dimension "d502" = 15
  dimension "d503" = 27.5
  dimension "d504" = 7.5
  dimension "d505" = 42.5
  dimension "d506" = 30
  dimension "d508" = 7.5
  dimension "d509" = 25
  dimension "d510" = 30
  dimension "d694" = 4.2
  dimension "d695" = 4.2
  dimension "d696" = 7.5
  dimension "d247" = 100
  dimension "d248" = 700
  dimension "d249" = 220
  dimension "d250" = 165
  dimension "d251" = 180
  dimension "d252" = 15
  dimension "d253" = 175
  dimension "d254" = 30
  dimension "d255" = 12
  dimension "d256" = 105
  dimension "d257" = 15
  dimension "d258" = 40
  dimension "d259" = 6
  dimension "d260" = 4
  dimension "d261" = 4
  dimension "d262" = 4
  dimension "d263" = 5
  dimension "d264" = 220
  dimension "d265" = 20
  dimension "d266" = 30
  dimension "d267" = 6
  dimension "d268" = 4
  dimension "d269" = 4
  dimension "d270" = 4
  dimension "d271" = 5
  dimension "d272" = 5
  dimension "d273" = 5
  dimension "d274" = 4.2
  dimension "d275" = 4.2
  dimension "d276" = 220
  dimension "d277" = 165
  dimension "d278" = 180
  dimension "d279" = 15
  dimension "d280" = 175
  dimension "d281" = 30
  dimension "d282" = 12
  dimension "d283" = 105
  dimension "d284" = 15
  dimension "d285" = 40
  dimension "d286" = 6
  dimension "d287" = 4
  dimension "d288" = 4
  dimension "d289" = 4
  dimension "d290" = 5
  dimension "d291" = 220
  dimension "d292" = 20
  dimension "d293" = 30
  dimension "d294" = 6
  dimension "d295" = 4
  dimension "d296" = 4
  dimension "d297" = 4
  dimension "d298" = 5
  dimension "d299" = 5
  dimension "d300" = 5
  dimension "d301" = 4.2
  dimension "d302" = 4.2
  dimension "d303" = 220
  dimension "d304" = 165
  dimension "d305" = 180
  dimension "d306" = 15
  dimension "d307" = 175
  dimension "d308" = 30
  dimension "d309" = 12
  dimension "d310" = 105
  dimension "d311" = 15
  dimension "d312" = 40
  dimension "d313" = 6
  dimension "d314" = 4
  dimension "d315" = 4
  dimension "d316" = 4
  dimension "d317" = 5
  dimension "d318" = 220
  dimension "d319" = 20
  dimension "d320" = 30
  dimension "d321" = 6
  dimension "d322" = 4
  dimension "d323" = 4
  dimension "d324" = 4
  dimension "d325" = 5
  dimension "d326" = 5
  dimension "d327" = 5
  dimension "d328" = 4.2
  dimension "d329" = 4.2
  dimension "d330" = 250
  dimension "d331" = 30
  dimension "d332" = 90
  dimension "d333" = 105
  dimension "d334" = 45
  dimension "d335" = 45
  dimension "d336" = 35
  dimension "d337" = 90
  dimension "d338" = 195
  dimension "d339" = 4.2
  dimension "d340" = 4.2
  dimension "d341" = 90
  dimension "d342" = 105
  dimension "d343" = 45
  dimension "d344" = 45
  dimension "d345" = 35
  dimension "d346" = 90
  dimension "d347" = 195
  dimension "d348" = 4.2
  dimension "d349" = 4.2
  dimension "d350" = 90
  dimension "d351" = 105
  dimension "d352" = 45
  dimension "d353" = 45
  dimension "d354" = 35
  dimension "d355" = 90
  dimension "d356" = 195
  dimension "d357" = 4.2
  dimension "d358" = 4.2
  dimension "d359" = 100
  dimension "d360" = 700
  dimension "d361" = 700
  dimension "d362" = 700
  dimension "d365" = 650
  dimension "d366" = 650
  dimension "d367" = 511.175
  dimension "d368" = 354.6391
  dimension "d369" = 511.175
  dimension "d370" = 75
  dimension "d371" = 354.6391
  dimension "d372" = 53.975
  dimension "d373" = 53.975
  dimension "d374" = 177.3195
  dimension "d375" = 69.85
  dimension "d376" = 7.5
  dimension "d377" = 7.5
  dimension "d520" = 2400
  dimension "d521" = 1800
  dimension "d522" = 700
  dimension "d523" = 1100
  dimension "d524" = 700
  dimension "d525" = 1100
  dimension "d526" = 700
  dimension "d527" = 1100
  dimension "d528" = 700
  dimension "d529" = 1100
  dimension "d530" = 700
  dimension "d531" = 1100
  dimension "d532" = 100
  dimension "d533" = 700
  dimension "d534" = 177.3195
  dimension "d535" = 177.3195
  dimension "d536" = 177.3195
  dimension "d537" = 177.3195
  dimension "d538" = 25.4
  dimension "d539" = 25.4
  dimension "d540" = 25.4
  dimension "d541" = 25.4
  dimension "d542" = 4.2
  dimension "d543" = 4.2
  dimension "d544" = 4.2
  dimension "d545" = 4.2
  dimension "d546" = 50.8
  dimension "d547" = 609.6
  dimension "d548" = 800
  dimension "d549" = 177.3195
  dimension "d550" = 177.3195
  dimension "d551" = 177.3195
  dimension "d552" = 177.3195
  dimension "d553" = 25.4
  dimension "d554" = 25.4
  dimension "d555" = 25.4
  dimension "d556" = 25.4
  dimension "d557" = 4.2
  dimension "d558" = 4.2
  dimension "d559" = 4.2
  dimension "d560" = 4.2
  dimension "d561" = 50.8
  dimension "d562" = 177.3195
  dimension "d563" = 177.3195
  dimension "d564" = 177.3195
  dimension "d565" = 177.3195
  dimension "d566" = 25.4
  dimension "d567" = 25.4
  dimension "d568" = 25.4
  dimension "d569" = 25.4
  dimension "d570" = 4.2
  dimension "d571" = 4.2
  dimension "d572" = 4.2
  dimension "d573" = 4.2
  dimension "d574" = 50.8
  dimension "d575" = 177.3195
  dimension "d576" = 177.3195
  dimension "d577" = 177.3195
  dimension "d578" = 177.3195
  dimension "d579" = 25.4
  dimension "d580" = 25.4
  dimension "d581" = 25.4
  dimension "d582" = 25.4
  dimension "d583" = 4.2
  dimension "d584" = 4.2
  dimension "d585" = 4.2
  dimension "d586" = 4.2
  dimension "d587" = 50.8
  dimension "d588" = 177.3195
  dimension "d589" = 177.3195
  dimension "d590" = 177.3195
  dimension "d591" = 177.3195
  dimension "d592" = 25.4
  dimension "d593" = 25.4
  dimension "d594" = 25.4
  dimension "d595" = 25.4
  dimension "d596" = 4.2
  dimension "d597" = 4.2
  dimension "d598" = 4.2
  dimension "d599" = 4.2
  dimension "d600" = 50.8
  dimension "d601" = 177.3195
  dimension "d602" = 177.3195
  dimension "d603" = 177.3195
  dimension "d604" = 177.3195
  dimension "d605" = 25.4
  dimension "d606" = 25.4
  dimension "d607" = 25.4
  dimension "d608" = 25.4
  dimension "d609" = 4.2
  dimension "d610" = 4.2
  dimension "d611" = 4.2
  dimension "d612" = 4.2
  dimension "d613" = 50.8
  dimension "d614" = 177.3195
  dimension "d615" = 177.3195
  dimension "d616" = 177.3195
  dimension "d617" = 177.3195
  dimension "d618" = 25.4
  dimension "d619" = 25.4
  dimension "d620" = 25.4
  dimension "d621" = 25.4
  dimension "d622" = 4.2
  dimension "d623" = 4.2
  dimension "d624" = 4.2
  dimension "d625" = 4.2
  dimension "d626" = 50.8
  dimension "d629" = 177.3195
  dimension "d630" = 177.3195
  dimension "d631" = 177.3195
  dimension "d632" = 177.3195
  dimension "d633" = 25.4
  dimension "d634" = 25.4
  dimension "d635" = 25.4
  dimension "d636" = 25.4
  dimension "d637" = 4.2
  dimension "d638" = 4.2
  dimension "d639" = 4.2
  dimension "d640" = 4.2
  dimension "d641" = 50.8
  dimension "d642" = 177.3195
  dimension "d643" = 177.3195
  dimension "d644" = 177.3195
  dimension "d645" = 177.3195
  dimension "d646" = 25.4
  dimension "d647" = 25.4
  dimension "d648" = 25.4
  dimension "d649" = 25.4
  dimension "d650" = 4.2
  dimension "d651" = 4.2
  dimension "d652" = 4.2
  dimension "d653" = 4.2
  dimension "d654" = 50.8
  dimension "d655" = 177.3195
  dimension "d656" = 177.3195
  dimension "d657" = 177.3195
  dimension "d658" = 177.3195
  dimension "d659" = 25.4
  dimension "d660" = 25.4
  dimension "d661" = 25.4
  dimension "d662" = 25.4
  dimension "d663" = 4.2
  dimension "d664" = 4.2
  dimension "d665" = 4.2
  dimension "d666" = 4.2
  dimension "d667" = 50.8
  dimension "d668" = 177.3195
  dimension "d669" = 177.3195
  dimension "d670" = 177.3195
  dimension "d671" = 177.3195
  dimension "d672" = 25.4
  dimension "d673" = 25.4
  dimension "d674" = 25.4
  dimension "d675" = 25.4
  dimension "d676" = 4.2
  dimension "d677" = 4.2
  dimension "d678" = 4.2